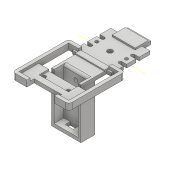
# Autodesk Inventor part: Intan_holder_v4_alt
Saved by Autodesk Inventor 2020 (Build 240168000, 168)
## iProperties
Created: 2018-08-30
Part Number: Intan_holder_v4_alt
Material: Generic
Document SubType Name: Modeling
Designer: huait
Density: 1 g/cm^3
Appearance: Default
Author: huait
Autodesk Inventor part; units mm, degrees
ref_plane "YZ Plane" through (0, 0, 0) normal (1, 0, 0) x (0, 1, 0)
ref_plane "XZ Plane" through (0, 0, 0) normal (0, 1, 0) x (-1, 0, 0)
ref_plane "XY Plane" through (0, 0, 0) normal (0, 0, 1) x (1, 0, 0)
sketch "Sketch1" plane through (0, 0, 0) normal (0, 0, 1) x (1, 0, 0)
  circle A0 centre (0, 0) radius 2.3
  line L0 (-9.1, -9.1) -> (9.1, 9.1) construction
  line L1 (9.1, -9.1) -> (-9.1, 9.1) construction
  circle A1 centre (9.1, 0) radius 1
  circle A2 centre (-9.1, 0) radius 1
  circle A3 centre (9.1, 3.8099) radius 1
  circle A4 centre (9.1, -3.81) radius 1
  circle A5 centre (-9.1, 3.8099) radius 1
  circle A6 centre (-9.1, -3.81) radius 1
  line L2 (-7, 17) -> (7, 17)
  line L3 (12, 11.5) -> (12, -12)
  line L4 (12, -12) -> (-12, -12)
  line L5 (-12, -12) -> (-12, 11.5)
  line L6 (-4.81, 9.1) -> (-9.1, 9.1)
  line L7 (9.1, 9.1) -> (4.81, 9.1)
  line L8 (9.1, 4.8099) -> (9.1, 9.1)
  line L9 (9.1, 1) -> (9.1, 2.8099)
  line L10 (9.1, -9.1) -> (9.1, -4.81)
  line L11 (9.1, -2.81) -> (9.1, -1)
  line L12 (4.81, -9.1) -> (9.1, -9.1)
  line L13 (-9.1, -9.1) -> (-4.81, -9.1)
  line L14 (-9.1, -4.81) -> (-9.1, -9.1)
  line L15 (-9.1, -1) -> (-9.1, -2.81)
  line L16 (-9.1, 9.1) -> (-9.1, 4.8099)
  line L17 (-9.1, 2.8099) -> (-9.1, 1)
  line L18 (4.81, 9.1) -> (-4.81, 9.1)
  line L19 (-4.81, -9.1) -> (4.81, -9.1)
  line L20 (-12, 11.5) -> (-7, 11.5)
  line L21 (-7, 11.5) -> (-7, 17)
  line L22 (12, 11.5) -> (7, 11.5)
  line L23 (7, 11.5) -> (7, 17)
  dimension "d0" = 18.2
  dimension "d1" = 18.2
  dimension "d6" = 2
  dimension "d7" = 2
  dimension "d10" = 4.6
  dimension "d11" = 2
  dimension "d12" = 2
  dimension "d15" = 2
  dimension "d16" = 2
  dimension "d17" = 3.8099
  dimension "d18" = 3.81
  dimension "d19" = 24
  dimension "d127" = 2.9
  dimension "d128" = 2.9
  dimension "d129" = 29
  dimension "d140" = 5
  dimension "d141" = 5
  dimension "d142" = 5.5
  constraints: 48 end point, 23 parallel, 12 point on circle, 11 perpendicular, 7 centre point, 6 collinear, 5 horizontal, 2 midpoint, 2 point on line, 1 coincident
  measures "d0" distance of L0.start L1.start
  measures "d1" distance of L1.start L0.end
  measures "d6" diameter of A1
  measures "d7" diameter of A2
  measures "d10" diameter of A0
  measures "d11" diameter of A3
  measures "d12" diameter of A4
  measures "d15" diameter of A5
  measures "d16" diameter of A6
  measures "d17" distance of A5.centre A2.centre
  measures "d18" distance of A2.centre A6.centre
  measures "d19" distance of L3.end L4.end
  measures "d127" distance between parallel lines of L4 L19
  measures "d128" distance between parallel lines of L14 L5
  measures "d129" distance between parallel lines of L2 L4
  measures "d140" distance of L3.start L22.end
  measures "d141" distance of L5.end L20.end
  measures "d142" distance of L2.start L20.end
extrude "Extrusion1" add sketch "Sketch1" along normal blind 2 contours A0 | A1 L11 A4 L10 L12 L19 L13 L14 A6 L15 A2 L17 A5 L16 L6 L18 L7 L8 A3 L9 | L2 L23 L22 L3 L4 L5 L20 L21
sketch "Sketch6" plane through (0, 0, 2) normal (0, 0, 1) x (1, 0, 0)
  circle A0 centre (-9.1, -3.81) radius 1 projected
  line L0 (-9.1, -4.81) -> (-13.3624, -4.81)
  line L1 (-13.3624, -4.81) -> (-13.3624, -2.81)
  line L2 (-13.3624, -2.81) -> (-9.1, -2.81)
  line L3 (-9.1, -2.81) -> (-9.1, -4.81)
  circle A1 centre (-9.1, 3.8099) radius 1 projected
  line L4 (-9.1, 2.8099) -> (-13.4787, 2.8099)
  line L5 (-13.4787, 2.8099) -> (-13.4787, 4.8099)
  line L6 (-13.4787, 4.8099) -> (-9.1, 4.8099)
  line L7 (-9.1, 4.8099) -> (-9.1, 2.8099)
  circle A2 centre (9.1, -3.81) radius 1 projected
  line L8 (9.1, -4.81) -> (13.9248, -4.81)
  line L9 (13.9248, -4.81) -> (13.9248, -2.81)
  line L10 (13.9248, -2.81) -> (9.1, -2.81)
  line L11 (9.1, -2.81) -> (9.1, -4.81)
  line L12 (9.1, 2.8099) -> (14.1963, 2.8099)
  line L13 (14.1963, 2.8099) -> (14.1963, 4.8099)
  line L14 (14.1963, 4.8099) -> (9.1, 4.8099)
  line L15 (9.1, 4.8099) -> (9.1, 2.8099)
  point P0 (0, 0)
  constraints: 32 end point, 8 parallel, 6 point on line, 4 horizontal, 4 perpendicular, 3 vertical alignment, 3 other
extrude "Extrusion5" cut sketch "Sketch6" against normal blind 40 contours L3 A0 | A0 L0 L1 L2 | L7 A1 | A1 L4 L5 L6 | A2 L11 | A2 L10 L9 L8 | L15 L14 L13 L12 picked at (-9.4117, -3.6918) picked at (-9.4117, 3.9281) picked at (9.1742, -3.485)
sketch "Sketch8" plane through (0, 0, 0) normal (1, 0, 0) x (0, 1, 0)
  line L0 (-12, 0) -> (-19.3, 0)
  line L1 (-19.3, 0) -> (-19.3, -28.65)
  line L2 (-19.3, -28.65) -> (-27.8, -28.65)
  line L3 (-27.8, -28.65) -> (-27.8, -26.65)
  line L4 (-27.8, -26.65) -> (-21.8, -26.65)
  line L5 (-21.8, -26.65) -> (-21.8, 2)
  line L6 (-21.8, 2) -> (-12, 2)
  line L7 (-12, 0) -> (-12, 2) projected
  line L8 (-12, 0) -> (-12, 2)
  line L9 (-13.3698, 2) -> (-13.3698, 2.7)
  line L10 (-13.3698, 2.7) -> (-10, 2.7)
  line L11 (-10, 2.7) -> (-10, 2)
  line L12 (-12, 2) -> (-10, 2)
  point P0 (0, 0)
  dimension "d49" = 2.5
  dimension "d50" = 7.3
  dimension "d51" = 28.65
  dimension "d52" = 2
  dimension "d53" = 2
  dimension "d54" = 0.7
  dimension "d57" = 6
  constraints: 24 end point, 7 perpendicular, 3 horizontal, 3 vertical, 1 point on line
  measures "d49" distance between parallel lines of L5 L1
  measures "d50" distance between parallel lines of L1 L7
  measures "d51" distance between parallel lines of L4 L6
  measures "d52" distance between parallel lines of L2 L4
  measures "d53" distance between parallel lines of L7 L11
  measures "d54" distance between parallel lines of L6 L10
  measures "d57" distance between parallel lines of L3 L5
extrude "Extrusion7" add sketch "Sketch8" along normal mid plane 18 separate body
sketch "Sketch9" plane through (-9, -21.8, -26.65) normal (0, -1, 0) x (1, 0, 0)
  line L0 (0, 0) -> (1.5, 0)
  line L1 (1.5, 0) -> (1.5, 28.65)
  line L2 (1.5, 28.65) -> (0, 28.65)
  line L3 (0, 28.65) -> (0, 0)
  line L4 (0, 0) -> (18, 0) projected
  line L5 (18, 0) -> (16.5, 0)
  line L6 (16.5, 0) -> (16.5, 28.65)
  line L7 (16.5, 28.65) -> (18, 28.65)
  line L8 (18, 28.65) -> (18, 0)
  line L9 (8, 28.65) -> (10, 28.65) projected
  line L10 (9, 28.65) -> (9, -2)
  line L11 (0, -2) -> (18, -2) projected
  line L12 (0, 28.65) -> (18, 28.65) projected
  point P0 (9, 26.65)
  dimension "d58" = 15
  constraints: 18 end point, 4 parallel, 2 horizontal, 2 midpoint, 2 perpendicular, 1 collinear, 1 point on line, 1 other
  measures "d58" distance between parallel lines of L6 L1
extrude "Extrusion8" add sketch "Sketch9" along normal blind 6 contours L3 L2 L1 L0 | L6 L7 L8 L4 bodies 2
sketch "Sketch10" plane through (-7.5, -29.8, -26.65) normal (0, 0, 1) x (1, 0, 0)
  line L0 (4, 4.8) -> (9, 4.8)
  line L1 (9, 4.8) -> (9, 8)
  line L2 (9, 8) -> (4, 8)
  line L3 (4, 8) -> (4, 4.8)
  line L4 (0, 8) -> (0, 2) projected
  line L5 (0, 8) -> (15, 8) projected
  point P0 (7.5, 29.8)
  point P1 (-2.5, 8)
  point P2 (17.5, 8)
  dimension "d63" = 4
  dimension "d64" = 5
  dimension "d65" = 3.2
  constraints: 8 end point, 2 parallel, 1 collinear, 1 horizontal, 1 perpendicular
  measures "d63" distance between parallel lines of L4 L3
  measures "d64" distance between parallel lines of L1 L3
  measures "d65" distance between parallel lines of L2 L0
extrude "Extrusion9" cut sketch "Sketch10" against normal blind 8 bodies 2
sketch "Sketch11" plane through (-7.5, -21.8, 2) normal (0, -1, 0) x (1, 0, 0)
  line L0 (0, -28.65) -> (0, 0) projected
  line L1 (0, -28.65) -> (15, -28.65) projected
  circle A0 centre (7.5, -5) radius 1.2
  line L2 (16.5, -2) -> (-1.5, -2) projected
  arc A1 (13.03, -25.49) -> (10.49, -25.49) centre (11.76, -25.49) ccw
  arc A2 (10.49, -26.09) -> (13.03, -26.09) centre (11.76, -26.09) ccw
  line L3 (10.49, -25.49) -> (10.49, -26.09)
  line L4 (13.03, -25.49) -> (13.03, -26.09)
  point P0 (7.5, -2)
  dimension "d74" = 2.4
  dimension "d75" = 3
  dimension "d119" = 2.54
  dimension "d120" = 2.54
  dimension "d123" = 11.76
  dimension "d124" = 3.16
  dimension "d125" = 0.6
  constraints: 4 end point, 4 point on circle, 3 centre point, 2 tangent, 1 parallel, 1 vertical
  measures "d74" diameter of A0
  measures "d75" distance from line of L2 A0.centre
  measures "d119" diameter of A1
  measures "d120" diameter of A2
  measures "d123" distance from line of L0 A1.centre
  measures "d124" distance from line of L1 A1.centre
  measures "d125" distance of L3.start L3.end
extrude "Extrusion10" cut sketch "Sketch11" against normal blind 8 bodies 2
fillet "Fillet1" radius 1.5 1 edges at (0, -21.8, 2)
sketch "Sketch12" plane through (0, 0, 2) normal (0, 0, 1) x (1, 0, 0)
  line L0 (15.25, -11) -> (15.25, -41.5)
  line L1 (-15.25, -41.5) -> (-15.25, -11)
  line L2 (-15.25, -11) -> (15.25, -41.5) construction
  line L3 (15.25, -11) -> (-15.25, -41.5) construction
  line L4 (-12, -12) -> (12, -12) projected
  line L5 (17.25, -9) -> (17.25, -43.5)
  line L6 (-17.25, -43.5) -> (-17.25, -9)
  line L7 (-8.45, -41.5) -> (-8.45, -43.5)
  line L8 (8.45, -41.5) -> (8.45, -43.5)
  line L9 (17.25, -43.5) -> (8.45, -43.5)
  line L10 (-8.45, -43.5) -> (-17.25, -43.5)
  line L11 (15.25, -41.5) -> (8.45, -41.5)
  line L12 (-8.45, -41.5) -> (-15.25, -41.5)
  line L13 (-9.2, -9) -> (-9.2, -11)
  line L14 (9.2, -9) -> (9.2, -11)
  line L15 (-9, -13.3698) -> (-9, -10) projected
  line L16 (9, -10) -> (9, -13.3698) projected
  line L17 (-17.25, -9) -> (-9.2, -9)
  line L18 (9.2, -9) -> (17.25, -9)
  line L19 (-15.25, -11) -> (-9.2, -11)
  line L20 (9.2, -11) -> (15.25, -11)
  point P0 (0, 0)
  point P1 (0, -26.25)
  dimension "d76" = 30.5
  dimension "d79" = 2
  dimension "d80" = 6.8
  dimension "d81" = 6.8
  dimension "d88" = 0.2
  dimension "d89" = 0.2
  constraints: 36 end point, 12 perpendicular, 10 parallel, 2 horizontal, 2 midpoint
  measures "d76" distance of L0.end L1.start
  measures "d79" distance between parallel lines of L6 L1
  measures "d80" distance between parallel lines of L1 L7
  measures "d81" distance between parallel lines of L0 L8
  measures "d88" distance between parallel lines of L13 L15
  measures "d89" distance between parallel lines of L14 L16
extrude "Extrusion11" add sketch "Sketch12" along normal blind 1.81 and the other way blind 2 bodies 1
sketch "Sketch13" plane through (0, 0, 0) normal (0, 0, -1) x (-1, 0, 0)
  line L0 (-15.25, -41.5) -> (-8.45, -41.5) projected
  line L1 (-15.25, -41.5) -> (-8.45, -41.5)
  line L2 (-8.45, -41.5) -> (-8.45, -39)
  line L3 (-8.45, -39) -> (-15.25, -39)
  line L4 (-15.25, -39) -> (-15.25, -41.5)
  line L5 (8.45, -41.5) -> (15.25, -41.5) projected
  line L6 (15.25, -41.5) -> (8.45, -41.5)
  line L7 (8.45, -41.5) -> (8.45, -39)
  line L8 (8.45, -39) -> (15.25, -39)
  line L9 (15.25, -39) -> (15.25, -41.5)
  line L10 (-15.25, -11) -> (-15.25, -41.5) projected
  line L11 (-15.25, -29.5) -> (15.25, -29.5)
  line L12 (15.25, -29.5) -> (15.25, -39)
  line L13 (15.25, -39) -> (-15.25, -39)
  line L14 (-15.25, -39) -> (-15.25, -29.5)
  point P0 (0, 0)
  dimension "d84" = 2.5
  dimension "d85" = 6.8
  dimension "d92" = 2.5
  dimension "d93" = 12
  constraints: 24 end point, 6 parallel, 3 horizontal, 3 perpendicular, 2 equal length, 1 point on line
  measures "d84" distance between parallel lines of L0 L3
  measures "d85" distance of L2.end L3.end
  measures "d92" distance between parallel lines of L5 L13
  measures "d93" distance between parallel lines of L5 L11
extrude "Extrusion12" add sketch "Sketch13" against normal blind 2.22 bodies 1
sketch "Sketch15" plane through (0, 0, 2.22) normal (0, 0, 1) x (1, 0, 0)
  line L0 (-9, -23.5) -> (9, -23.5)
  line L1 (9, -23.5) -> (9, -35.5)
  line L2 (9, -35.5) -> (-9, -35.5)
  line L3 (-9, -35.5) -> (-9, -23.5)
  line L4 (15.25, -29.5) -> (-15.25, -29.5) projected
  line L5 (-9, -23.5) -> (9, -35.5) construction
  line L6 (9, -23.5) -> (-9, -35.5) construction
  line L7 (15.25, -41.5) -> (8.45, -41.5) projected
  point P0 (0, 0)
  point P1 (0, -29.5)
  dimension "d94" = 18
  dimension "d95" = 6
  constraints: 12 end point, 3 midpoint, 2 parallel, 1 horizontal, 1 perpendicular
  measures "d94" distance between parallel lines of L1 L3
  measures "d95" distance between parallel lines of L7 L2
extrude "Extrusion13" cut sketch "Sketch15" against normal blind 1 bodies 1
sketch "Sketch17" plane through (0, 0, 0) normal (0, 0, -1) x (-1, 0, 0)
  circle A0 centre (-7.5, -34) radius 1.2
  circle A1 centre (7.5, -34) radius 1.2
  line L0 (-8.45, -39) -> (8.45, -39) projected
  line L1 (15.25, -29.5) -> (-15.25, -29.5) projected
  line L2 (8.45, -39) -> (-8.45, -39) construction
  line L3 (0, -39) -> (0, -29.5) construction
  point P0 (0, 0)
  dimension "d115" = 2.4
  dimension "d151" = 7.5
  dimension "d152" = 7.5
  dimension "d153" = 5
  dimension "d154" = 5
  constraints: 2 centre point, 2 end point, 2 midpoint, 1 equal radius
  measures "d115" diameter of A0
  measures "d151" distance from line of L3 A0.centre
  measures "d152" distance from line of L3 A1.centre
  measures "d153" distance from line of L0 A1.centre
  measures "d154" distance from line of L0 A0.centre
extrude "Extrusion15" cut sketch "Sketch17" against normal blind 12 bodies 1
fillet "Fillet2" radius 2 4 edges at (-17.25, -43.5, 1.905) (17.25, -43.5, 1.905) (17.25, -9, 1.905) (-17.25, -9, 1.905)
sketch "Sketch18" plane through (0, 0, 2) normal (0, 0, 1) x (1, 0, 0)
  circle A0 centre (0, -1) radius 1.575
  line L0 (-9, -10) -> (9, -10) construction
  point P0 (0, 0)
  dimension "d131" = 3.15
  dimension "d175" = 9
  constraints: 1 centre point
  measures "d131" diameter of A0
  measures "d175" distance from line of L0 A0.centre
extrude "Extrusion16" cut sketch "Sketch18" against normal blind 10 bodies 1
sketch "Sketch26" plane through (0, 0, 2) normal (0, 0, 1) x (1, 0, 0)
  line L0 (-7, 7.38) -> (7, 7.38)
  line L1 (7, 7.38) -> (7, 15.43)
  line L2 (7, 15.43) -> (-7, 15.43)
  line L3 (-7, 15.43) -> (-7, 7.38)
  circle A0 centre (0, -1) radius 1.575 construction
  point P0 (0, 0)
  dimension "d176" = 8.38
  dimension "d177" = 8.05
  constraints: 8 end point, 2 parallel, 1 horizontal, 1 perpendicular
  measures "d176" distance from line of A0.centre L0
  measures "d177" distance between parallel lines of L2 L0
extrude "Extrusion24" add sketch "Sketch26" along normal blind 1 bodies 1
sketch "Sketch21" plane through (0, 0, 3.81) normal (0, 0, 1) x (1, 0, 0)
  arc A0 (-15.25, -9) -> (-17.25, -11) centre (-15.25, -11) ccw projected
  line L0 (-17.25, -11) -> (-17.25, -41.5) projected
  arc A1 (-17.25, -41.5) -> (-15.25, -43.5) centre (-15.25, -41.5) ccw projected
  line L1 (-15.25, -43.5) -> (-8.45, -43.5) projected
  line L2 (-8.45, -43.5) -> (-8.45, -41.5) projected
  line L3 (-8.45, -41.5) -> (-15.25, -41.5) projected
  line L4 (-15.25, -41.5) -> (-15.25, -11) projected
  line L5 (-15.25, -11) -> (-9.2, -11) projected
  line L6 (-9.2, -11) -> (-9.2, -9) projected
  line L7 (-9.2, -9) -> (-15.25, -9) projected
  arc A2 (17.25, -11) -> (15.25, -9) centre (15.25, -11) ccw projected
  line L8 (15.25, -9) -> (9.2, -9) projected
  line L9 (9.2, -9) -> (9.2, -11) projected
  line L10 (9.2, -11) -> (15.25, -11) projected
  line L11 (15.25, -11) -> (15.25, -41.5) projected
  line L12 (15.25, -41.5) -> (8.45, -41.5) projected
  line L13 (8.45, -41.5) -> (8.45, -43.5) projected
  line L14 (8.45, -43.5) -> (15.25, -43.5) projected
  arc A3 (15.25, -43.5) -> (17.25, -41.5) centre (15.25, -41.5) ccw projected
  line L15 (17.25, -41.5) -> (17.25, -11) projected
  line L16 (-8.45, -43.5) -> (-8.45, -39) projected
  line L17 (-8.45, -43.5) -> (8.45, -43.5)
  line L18 (7.15, -9) -> (-7.15, -9)
  line L19 (-15.25, -41.5) -> (-15.25, -11) projected
  line L20 (-15.25, -41.5) -> (-15.25, -11)
  line L21 (9.2, -11) -> (15.25, -11) projected
  line L22 (-15.25, -11) -> (15.25, -11)
  line L23 (15.25, -11) -> (15.25, -41.5) projected
  line L24 (15.25, -11) -> (15.25, -41.5)
  line L25 (-15.25, -41.5) -> (15.25, -41.5)
  line L26 (15.25, -9) -> (9.2, -9) projected
  line L27 (12, -9) -> (12, 1)
  line L28 (7.15, 1) -> (7.15, -9)
  line L29 (-7.15, 1) -> (-7.15, -9)
  line L30 (7, 5.1664) -> (7, 17) projected
  line L31 (-7, 17) -> (-7, 5.1664) projected
  line L32 (-12, -4.81) -> (-12, -9) projected
  line L33 (-12, -9) -> (-12, 1)
  line L34 (-12, 1) -> (-7.15, 1)
  line L35 (7.15, 1) -> (12, 1)
  point P0 (0, 0)
  dimension "d161" = 0.15
  dimension "d162" = 0.15
  dimension "d163" = 10
  constraints: 24 end point, 4 collinear, 3 perpendicular, 3 vertical, 2 horizontal
  measures "d161" distance between parallel lines of L30 L28
  measures "d162" distance between parallel lines of L31 L29
  measures "d163" distance of L32.end L33.end
sketch "Sketch22" plane through (0, 0, 3.81) normal (0, 0, -1) x (-1, 0, 0)
  arc A0 (17.25, -11) -> (15.25, -9) centre (15.25, -11) ccw projected
  line L0 (12, -9) -> (15.25, -9) projected
  line L1 (-7.15, -9) -> (7.15, -9) projected
  line L2 (-15.25, -9) -> (-12, -9) projected
  arc A1 (-15.25, -9) -> (-17.25, -11) centre (-15.25, -11) ccw projected
  line L3 (-17.25, -41.5) -> (-17.25, -11) projected
  arc A2 (-17.25, -41.5) -> (-15.25, -43.5) centre (-15.25, -41.5) ccw projected
  line L4 (-8.45, -43.5) -> (-15.25, -43.5) projected
  line L5 (-8.45, -41.5) -> (-8.45, -43.5) projected
  line L6 (-15.25, -41.5) -> (-8.45, -41.5) projected
  line L7 (15.25, -11) -> (-15.25, -11) projected
  line L8 (15.25, -41.5) -> (15.25, -11) projected
  line L9 (8.45, -41.5) -> (15.25, -41.5) projected
  line L10 (8.45, -43.5) -> (8.45, -41.5) projected
  line L11 (15.25, -43.5) -> (8.45, -43.5) projected
  arc A3 (15.25, -43.5) -> (17.25, -41.5) centre (15.25, -41.5) ccw projected
  line L12 (17.25, -11) -> (17.25, -41.5) projected
  line L13 (7.15, -9) -> (7.15, 1) projected
  line L14 (-7.15, 1) -> (-7.15, -9) projected
  line L15 (-12, -9) -> (-12, 1) projected
  line L16 (-15.25, -11) -> (-15.25, -41.5) projected
  line L17 (-12, -9) -> (-7.15, -9)
  line L18 (12, -9) -> (7.15, -9)
  line L19 (12, 1) -> (12, -9) projected
  line L20 (7.15, 1) -> (12, 1) projected
  line L21 (-12, 1) -> (-7.15, 1) projected
  constraints: 4 end point, 1 collinear, 1 horizontal
sketch "Sketch23" plane through (0, 0, 5.81) normal (0, 0, 1) x (1, 0, 0)
  line L0 (-8.45, -43.5) -> (-8.45, -41.5) projected
  line L1 (-8.45, -41.5) -> (-15.25, -41.5) projected
  line L2 (-15.25, -41.5) -> (-15.25, -11) projected
  line L3 (-15.25, -11) -> (15.25, -11) projected
  line L4 (15.25, -11) -> (15.25, -41.5) projected
  line L5 (15.25, -41.5) -> (8.45, -41.5) projected
  line L6 (8.45, -41.5) -> (8.45, -43.5) projected
  line L7 (8.45, -43.5) -> (15.25, -43.5) projected
  arc A0 (15.25, -43.5) -> (17.25, -41.5) centre (15.25, -41.5) ccw projected
  line L8 (17.25, -41.5) -> (17.25, -11) projected
  arc A1 (17.25, -11) -> (15.25, -9) centre (15.25, -11) ccw projected
  line L9 (15.25, -9) -> (12, -9) projected
  line L10 (12, -9) -> (12, 1) projected
  line L11 (12, 1) -> (7.15, 1) projected
  line L12 (7.15, 1) -> (7.15, -9) projected
  line L13 (7.15, -9) -> (-7.15, -9) projected
  line L14 (-7.15, -9) -> (-7.15, 1) projected
  line L15 (-7.15, 1) -> (-12, 1) projected
  line L16 (-12, 1) -> (-12, -9) projected
  line L17 (-12, -9) -> (-15.25, -9) projected
  arc A2 (-15.25, -9) -> (-17.25, -11) centre (-15.25, -11) ccw projected
  line L18 (-17.25, -11) -> (-17.25, -41.5) projected
  arc A3 (-17.25, -41.5) -> (-15.25, -43.5) centre (-15.25, -41.5) ccw projected
  line L19 (-15.25, -43.5) -> (-8.45, -43.5) projected
  line L20 (-8.45, -43.5) -> (8.45, -43.5)
  line L21 (-12, -9) -> (-12, -4.81) projected
  line L22 (-12, -9) -> (12, -9)
  line L23 (15.25, -9) -> (9.2, -9) projected
  line L24 (-8.45, -41.5) -> (8.45, -41.5)
  point P0 (0, 0)
  constraints: 6 end point, 2 horizontal, 1 collinear
sketch "Sketch24" plane through (0, 0, 10.81) normal (0, 0, 1) x (1, 0, 0)
  line L0 (15.25, -41.5) -> (-15.25, -41.5) projected
  line L1 (-15.25, -41.5) -> (-15.25, -11) projected
  line L2 (-15.25, -11) -> (15.25, -11) projected
  line L3 (15.25, -11) -> (15.25, -41.5) projected
  line L4 (-15.25, -43.5) -> (15.25, -43.5) projected
  arc A0 (15.25, -43.5) -> (17.25, -41.5) centre (15.25, -41.5) ccw projected
  line L5 (17.25, -41.5) -> (17.25, -11) projected
  arc A1 (17.25, -11) -> (15.25, -9) centre (15.25, -11) ccw projected
  line L6 (15.25, -9) -> (-15.25, -9) projected
  arc A2 (-15.25, -9) -> (-17.25, -11) centre (-15.25, -11) ccw projected
  line L7 (-17.25, -11) -> (-17.25, -41.5) projected
  arc A3 (-17.25, -41.5) -> (-15.25, -43.5) centre (-15.25, -41.5) ccw projected
  point P0 (0, 0)
sketch "Sketch25" plane through (15.25, -11, 2) normal (0, 0, -1) x (-1, 0, 0)
  circle A0 centre (5.25, 7.19) radius 1
  line L0 (6.15, 8.19) -> (3.25, 8.19) projected
  circle A1 centre (25.25, 7.19) radius 1
  line L1 (27.25, 8.19) -> (24.35, 8.19) projected
  line L2 (24.35, 6.19) -> (27.25, 6.19) projected
  line L3 (25.25, 6.19) -> (27.25, 6.19)
  line L4 (27.25, 6.19) -> (27.25, 8.19)
  line L5 (5.25, 8.19) -> (3.25, 8.19)
  line L6 (3.25, 6.19) -> (5.25, 6.19)
  line L7 (3.25, 12) -> (3.25, 2) projected
  line L8 (3.25, 6.19) -> (3.25, 8.19)
  line L9 (25.25, 8.19) -> (27.25, 8.19)
  point P0 (15.25, 11)
  dimension "d168" = 2
  dimension "d169" = 2
  dimension "d170" = 2
  dimension "d171" = 2
  constraints: 12 end point, 4 point on circle, 4 tangent, 3 point on line, 2 centre point, 2 collinear, 2 horizontal, 2 perpendicular, 1 vertical
  measures "d168" diameter of A0
  measures "d169" diameter of A1
  measures "d170" distance of L3.start L2.end
  measures "d171" distance of L6.start L6.end
body "Solid1"
body "Solid2"
body "Solid3"
body "Solid4"
